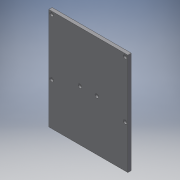
# Autodesk Inventor part: A0005
Saved by Autodesk Inventor 2017 (Build 210142000, 142)
## iProperties
Part Number: A0005
Material: 一般
Document SubType Name: Modeling
Designer: lygfy
Density: 1 g/cm^3
Appearance: 預設
Author: lygfy
Autodesk Inventor part; units mm, degrees
ref_plane "YZ Plane" through (0, 0, 0) normal (1, 0, 0) x (0, 1, 0)
ref_plane "XZ Plane" through (0, 0, 0) normal (0, 1, 0) x (-1, 0, 0)
ref_plane "XY Plane" through (0, 0, 0) normal (0, 0, 1) x (1, 0, 0)
sketch "草圖1" plane through (0, 0, 0) normal (0, 1, 0) x (-1, 0, 0)
  line L0 (70, -124.9774) -> (-70, -124.9774)
  line L1 (-70, -124.9774) -> (-70, 55.0226)
  line L2 (-70, 55.0226) -> (70, 55.0226)
  line L3 (70, 55.0226) -> (70, -124.9774)
  point P0 (0, 0)
  point P1 (0, 55.0226)
  dimension "d0" = 140
  dimension "d1" = 180
  constraints: 8 end point, 2 parallel, 1 horizontal, 1 midpoint, 1 perpendicular, 1 vertical alignment
  measures "d0" distance of L1.end L2.end
  measures "d1" distance of L0.end L1.end
extrude "擠出1" add sketch "草圖1" along normal blind 6
sketch "草圖2" plane through (0, 0, 0) normal (0, -1, 0) x (1, 0, 0)
  line L0 (-65, 50.0226) -> (65, 50.0226)
  line L1 (65, 50.0226) -> (65, -49.9774)
  line L2 (65, -49.9774) -> (-65, -49.9774)
  line L3 (-65, -49.9774) -> (-65, 50.0226)
  line L4 (70, 55.0226) -> (-70, 55.0226) projected
  line L5 (15, -54.9774) -> (-15, -54.9774)
  point P0 (0, 0)
  point P1 (0, 50.0226)
  point P2 (0, -54.9774)
  dimension "d18" = 130
  dimension "d19" = 100
  dimension "d20" = 5
  dimension "d21" = 30
  dimension "d22" = 110
  constraints: 10 end point, 2 horizontal, 2 midpoint, 2 parallel, 2 vertical alignment, 1 perpendicular
  measures "d18" distance of L0.start L0.end
  measures "d19" distance of L0.end L1.end
  measures "d20" distance between parallel lines of L0 L4
  measures "d21" distance of L5.start L5.end
  measures "d22" distance between parallel lines of L5 L4
hole "孔1" at (65, 0, 50.0226) at (65, 0, -49.9774) at (-65, 0, -49.9774) at (-65, 0, 50.0226) at (15, 0, -54.9774) at (-15, 0, -54.9774) direction (0, 1, 0) diameter 3.3 end through all counterbore diameter 6.5 counterbore depth 3.3
sketch "草圖3" plane through (0, 6, 0) normal (0, 1, 0) x (1, 0, 0)
  circle A0 centre (0, 94.9774) radius 22.5
  line L0 (-70, -55.0226) -> (70, -55.0226) projected
  point P0 (0, 0)
  dimension "d15" = 45
  dimension "d23" = 150
  constraints: 1 centre point, 1 vertical alignment
  measures "d15" diameter of A0
  measures "d23" distance from line of L0 A0.centre
extrude "擠出2" cut sketch "草圖3" against normal blind 0.1
